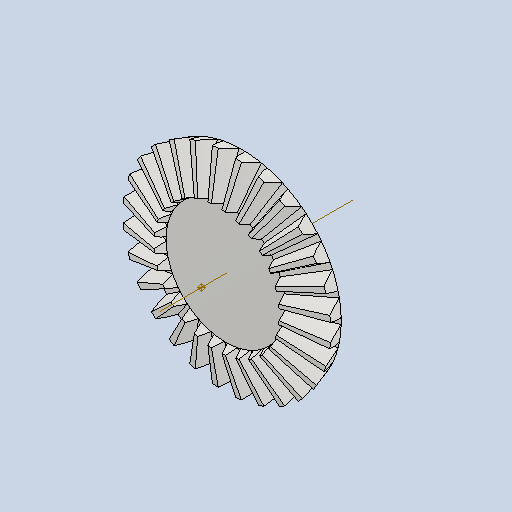
# Autodesk Inventor part: 베벨 기어2
Saved by Autodesk Inventor 2025.3 (Build 293356030, 356C)
## iProperties
Created: 2025-11-17
Part Number: 베벨 기어2
Material: Steel, Mild
Document SubType Name: Modeling
Designer: MSI
Categories: <?xml version="1.0" encoding="UTF-16"?> <MemberInstance><Categories><FamilyTemplate><FamilyTemplateParameter ValueType="xs:double" Id="1" ObjectReferenceKey="da_z" ObjectType="kUserParameterObject"/><FamilyTemplateParameter ValueType="xs:double" Id="2" ObjectReferenceKey="da_b" ObjectType="kUserParameterObject"/><FamilyTemplateParameter ValueType="xs:double" Id="3" ObjectReferenceKey="da_beta" ObjectType="kUserParameterObject"/><FamilyTemplateParameter ValueType="xs:double" Id="4" ObjectReferenceKey="da_dae" ObjectType="kUserParameterObject"/><FamilyTemplateParameter ValueType="xs:double" Id="5" ObjectReferenceKey="da_ve" ObjectType="kUserParameterObject"/><FamilyTemplateParameter ValueType="xs:double" Id="6" ObjectReferenceKey="da_omega" ObjectType="kUserParameterObject"/><FamilyTemplateParameter ValueType="xs:string" Id="7" ObjectReferenceKey="EAIAABAAAAAAHwAAAAAAAIAAAAAAAAAA" ObjectType="83914240" SubObjectId="SurfaceGeometry"/></FamilyTemplate><ParamToTemplateMap><ParamToTemplate CategoryParameter="//CategoryParameter[@InternalName='046C89C9-8512-4d59-83FE-43B91F4F132A']" TemplateParameter="1"/><ParamToTemplate CategoryParameter="//CategoryParameter[@InternalName='2552DF32-E462-4b46-AEBF-C6C7768E72AC']" TemplateParameter="2"/><ParamToTemplate CategoryParameter="//CategoryParameter[@InternalName='C9EE641D-15FC-4fae-A226-E94C4372FDD7']" TemplateParameter="3"/><ParamToTemplate><ParamToTemplate CategoryParameter="//CategoryParameter[@InternalName='00B6519A-459B-49c7-AD84-2E56D39A5744']" ConstantValue="-0.000000"/></ParamToTemplate><ParamToTemplate><ParamToTemplate CategoryParameter="//CategoryParameter[@InternalName='04B31F0E-C7A6-4894-AA32-9629BEFACF47']" ConstantValue="1.000000"/></ParamToTemplate><ParamToTemplate><ParamToTemplate CategoryParameter="//CategoryParameter[@InternalName='43CBEC2E-7847-49e7-A936-2F7889FCB2D9']" ConstantValue="0.200000"/></ParamToTemplate><ParamToTemplate><ParamToTemplate CategoryParameter="//CategoryParameter[@InternalName='B1EFC894-105D-4ebd-86BF-FA20ED196853']" ConstantValue="0.300000"/></ParamToTemplate><ParamToTemplate><ParamToTemplate CategoryParameter="//CategoryParameter[@InternalName='51175063-3D10-4879-93E8-6246FE8B403D']" ConstantValue="2060000000.000000"/></ParamToTemplate><ParamToTemplate><ParamToTemplate CategoryParameter="//CategoryParameter[@InternalName='A3A52E27-4454-46a9-B0BD-C932399B70AF']" ConstantValue="0.300000"/></ParamToTemplate><ParamToTemplate CategoryParameter="//CategoryParameter[@InternalName='2A200944-5A8C-41ca-B96E-8520D2E510F1']" TemplateParameter="4"/><ParamToTemplate><ParamToTemplate CategoryParameter="//CategoryParameter[@InternalName='1A637F62-92C8-44bc-B81F-10802510B579']" ConstantValue="3.445963"/></ParamToTemplate><ParamToTemplate CategoryParameter="//CategoryParameter[@InternalName='B52DD4BE-6863-48fb-BF58-89EF6F9EC65C']" TemplateParameter="5"/><ParamToTemplate><ParamToTemplate CategoryParameter="//CategoryParameter[@InternalName='3956BFF2-84D2-457d-93C2-9B0613DEBA67']" ConstantValue="0.427309"/></ParamToTemplate><ParamToTemplate CategoryParameter="//CategoryParameter[@InternalName='739CFA02-461B-4bf8-8049-181FCAD8B28F']" TemplateParameter="6"/><ParamToTemplate><ParamToTemplate CategoryParameter="//CategoryParameter[@InternalName='A27E999F-E2CE-4481-8A2A-EBF499C4C3C5']" ConstantValue="-0.000000"/></ParamToTemplate><ParamToTemplate><ParamToTemplate CategoryParameter="//CategoryParameter[@InternalName='9E1B4470-B2D3-4ff1-B813-535BB4CDF51A']" ConstantValue="3520000.000000"/></ParamToTemplate><ParamToTemplate><ParamToTemplate CategoryParameter="//CategoryParameter[@InternalName='F8452263-BFF6-458c-9FB1-07C4B99E95CD']" ConstantValue="11400000.000000"/></ParamToTemplate><ParamToTemplate><ParamToTemplate CategoryParameter="//CategoryParameter[@InternalName='3E3BB259-FD49-497f-8171-6EBC954A3479']" ConstantValue="2.000000"/></ParamToTemplate><ParamToTemplate CategoryParameter="//CategoryParameter[@InternalName='27C3BAF2-7550-4e4b-AE2C-0DB134B7D9B7']" TemplateParameter="7"/></ParamToTemplateMap><Category DisplayName="Gear" InternalName="DC85795E-93AB-48d5-8EEE-5A27447B64BD" Mnemonic="Gear"><CategoryParameter DisplayName="z" InternalName="046C89C9-8512-4d59-83FE-43B91F4F132A" Mnemonic="z"/><CategoryParameter DisplayName="b" InternalName="2552DF32-E462-4b46-AEBF-C6C7768E72AC" Mnemonic="b"/><CategoryParameter DisplayName="||b|" InternalName="C9EE641D-15FC-4fae-A226-E94C4372FDD7" Mnemonic="beta"/><CategoryParameter DisplayName="x" InternalName="00B6519A-459B-49c7-AD84-2E56D39A5744" Mnemonic="x"/><CategoryParameter DisplayName="a*" InternalName="04B31F0E-C7A6-4894-AA32-9629BEFACF47" Mnemonic="a"/><CategoryParameter DisplayName="c*" InternalName="43CBEC2E-7847-49e7-A936-2F7889FCB2D9" Mnemonic="c"/><CategoryParameter DisplayName="r|.f|*" InternalName="B1EFC894-105D-4ebd-86BF-FA20ED196853" Mnemonic="rf"/><CategoryParameter DisplayName="E" InternalName="51175063-3D10-4879-93E8-6246FE8B403D" Mnemonic="E"/><CategoryParameter DisplayName="||m|" InternalName="A3A52E27-4454-46a9-B0BD-C932399B70AF" Mnemonic="mi"/><Category DisplayName="BevelGear" InternalName="0C98F69A-0C2B-4791-B2FE-7691BB227E77" Mnemonic="BevelGear"><CategoryParameter DisplayName="d|.ae|" InternalName="2A200944-5A8C-41ca-B96E-8520D2E510F1" Mnemonic="dae"/><CategoryParameter DisplayName="d|.ai|" InternalName="1A637F62-92C8-44bc-B81F-10802510B579" Mnemonic="dai"/><CategoryParameter DisplayName="A|.e|" InternalName="B52DD4BE-6863-48fb-BF58-89EF6F9EC65C" Mnemonic="ve"/><CategoryParameter DisplayName="A|.i|" InternalName="3956BFF2-84D2-457d-93C2-9B0613DEBA67" Mnemonic="vi"/><CategoryParameter DisplayName="||S|" InternalName="739CFA02-461B-4bf8-8049-181FCAD8B28F" Mnemonic="omega"/><CategoryParameter DisplayName="x|.t|" InternalName="A27E999F-E2CE-4481-8A2A-EBF499C4C3C5" Mnemonic="xt"/><CategoryParameter DisplayName="||s||.Flim|" InternalName="9E1B4470-B2D3-4ff1-B813-535BB4CDF51A" Mnemonic="sFlim"/><CategoryParameter DisplayName="||s||.Hlim|" InternalName="F8452263-BFF6-458c-9FB1-07C4B99E95CD" Mnemonic="sHlim"/><CategoryParameter DisplayName="유형" InternalName="3E3BB259-FD49-497f-8171-6EBC954A3479" Mnemonic="type"/><CategoryParameter DisplayName="PitchDiameter" InternalName="27C3BAF2-7550-4e4b-AE2C-0DB134B7D9B7" Mnemonic="IDS_PITCHDIAM"/></Category></Category></Categories></MemberInstance>
Mass: 60.9118 g
Surface Area: 34.3074 cm^2
Volume: 7.7496 cm^3
Density: 7.86 g/cm^3
Appearance: Steel
CustomPartVersion: 1
Author: MSI
Autodesk Inventor part; units mm, degrees
ref_plane "메쉬 평면2" through (0, 0, 0) normal (0.9937122, 0.1119645, 0) x (0, 0, 1)
sketch "톱니 본체 스케치" plane through (0, 0, 0) normal (1, 0, 0) x (0, 1, 0)
  line L0 (0, 0) -> (27.265578, -11.284869) construction
  line L1 (27.265578, -11.284869) -> (28.612018, -7.095943)
  line L2 (28.612018, -7.095943) -> (0, 0) construction
  line L3 (28, -9) -> (0, 0) construction
  line L4 (16.419006, -6.795613) -> (17.229816, -4.273092)
  line L5 (27.265578, -11.284869) -> (16.419006, -6.795613)
  line L6 (28.612018, -7.095943) -> (17.229816, -4.273092)
  line L7 (0, -39.386751) -> (0, 6.564458)
  line L8 (0, -9) -> (28.612018, -9) construction
  dimension "d0" = 56
  dimension "d1" = 54.53116
  dimension "d2" = 57.22404
  dimension "d3" = 11.7
  dimension "d4" = 7.09594
  constraints: 16 end point, 4 point on line, 3 perpendicular, 2 collinear, 1 horizontal alignment, 1 vertical alignment
  measures "d0" diameter of L3.start L7
  measures "d1" diameter of L0.end L7
  measures "d2" diameter of L1.end L7
  measures "d3" distance between parallel lines of L1 L4
  measures "d4" vertical distance of L1.end L0.start
revolve "톱니 본체" add sketch "톱니 본체 스케치" angle 360 about axis through (0, 0, 0) along (0, 0, 1)
ref_plane "톱니 평면" through (0, 28, -9) normal (0, -0.9520286, 0.3060092) x (1, 0, 0)
sketch "시작 스케치" plane through (0, 28, -9) normal (0, -0.9520286, 0.3060092) x (1, 0, 0)
  line L0 (0, -23.505131) -> (0, 10.644758)
  arc A0 (-0.660229, -2.927998) -> (-3.024625, 3.271749) centre (-31.571304, -11.165819) ccw
  arc A1 (3.024625, 3.271749) -> (0.660229, -2.927998) centre (31.571304, -11.165819) ccw
  line L1 (-0.660229, -2.927998) -> (0.660229, -2.927998)
  arc A2 (3.024625, 3.271749) -> (-3.024625, 3.271749) centre (0, -91.500521) ccw
  dimension "d7" = 31.98994
  dimension "d8" = 31.5713
  dimension "d9" = 80.3347
  dimension "d57" = 94.82052
  dimension "d58" = 88.57252
  constraints: 6 point on circle, 3 centre point, 3 symmetric about line, 2 end point, 1 coincident, 1 perpendicular, 1 other
  measures "d7" radius of A0
  measures "d8" horizontal distance of point (0, -91.501) A0.centre
  measures "d9" vertical distance of point (0, -91.501) A0.centre
  measures "d57" radius of A2
  measures "d58" distance from line of A2.centre L1
ref_plane "끝 평면" through (0, 16.65182, -5.352371) normal (0, -0.9520286, 0.3060092) x (1, 0, 0)
sketch "끝 스케치" plane through (0, 16.65182, -5.352371) normal (0, -0.9520286, 0.3060092) x (1, 0, 0)
  line L0 (0, -15.35404) -> (0, 6.953444)
  arc A0 (-0.392643, -1.741305) -> (-1.798768, 1.945734) centre (-18.775702, -6.640401) ccw
  arc A1 (1.798768, 1.945734) -> (0.392643, -1.741305) centre (18.775702, -6.640401) ccw
  line L1 (-0.392643, -1.741305) -> (0.392643, -1.741305)
  arc A2 (1.798768, 1.945734) -> (-1.798768, 1.945734) centre (0, -54.416078) ccw
  dimension "d12" = 19.02467
  dimension "d15" = 18.7757
  dimension "d16" = 47.77568
  dimension "d59" = 56.39051
  dimension "d60" = 52.67477
  constraints: 6 point on circle, 3 centre point, 3 symmetric about line, 2 end point, 1 coincident, 1 other
  measures "d12" radius of A0
  measures "d15" horizontal distance of A0.centre point (0, -54.416)
  measures "d16" vertical distance of A0.centre point (0, -54.416)
  measures "d59" radius of A2
  measures "d60" distance from line of A2.centre L1
loft "Loft" cut profiles "시작 스케치", "끝 스케치"
pattern_circular "Circular Pattern" count 28 over 360 about axis through (0, 0, 0) along (0, 0, 1) of "Loft"
sketch3d "3D 스케치 오른쪽"
ref_plane "끝 평면 오른쪽" through (-3.200744, 16.341307, -5.352371) normal (0.182995, -0.9342758, 0.3060092) x (0.9813527, 0.1922159, 0)
sketch "끝 스케치 오른쪽" plane through (-3.200744, 16.341307, -5.352371) normal (0.182995, -0.9342758, 0.3060092) x (0.9813527, 0.1922159, 0)
  arc A0 (-0.392643, -1.741305) -> (-1.798768, 1.945734) centre (-18.775702, -6.640401) ccw
  line L0 (0, -67.117491) -> (0, 16.468068)
  arc A1 (1.798768, 1.945734) -> (0.392643, -1.741305) centre (18.775702, -6.640401) ccw
  line L1 (-0.392643, -1.741305) -> (0.392643, -1.741305)
  arc A2 (1.798768, 1.945734) -> (-1.798768, 1.945734) centre (0, -54.416078) ccw
  dimension "d70" = 18.7757
  dimension "d71" = 47.77568
  dimension "d72" = 19.02467
  dimension "d73" = 52.67477
  dimension "d74" = 56.39051
  constraints: 6 point on circle, 3 centre point, 3 symmetric about line, 2 end point, 1 coincident, 1 perpendicular, 1 other
  measures "d70" horizontal distance of A2.centre A0.centre
  measures "d71" vertical distance of point (0, -54.416) A0.centre
  measures "d72" radius of A0
  measures "d73" distance from line of point (0, -54.416) L1
  measures "d74" radius of A2
feature "로프트 오른쪽" [suppressed]
pattern_circular "원형 패턴 오른쪽" [suppressed]
sketch3d "3D 스케치 왼쪽"
ref_plane "끝 평면 왼쪽" through (3.32113, 16.341307, -5.46163) normal (-0.1892704, -0.9312872, 0.311257) x (0.9799662, -0.1991637, 0)
sketch "끝 스케치 왼쪽" plane through (3.32113, 16.341307, -5.46163) normal (-0.1892704, -0.9312872, 0.311257) x (0.9799662, -0.1991637, 0)
  line L0 (0, -68.172924) -> (0, 17.623134)
  arc A0 (-0.392643, -1.643977) -> (-1.798768, 2.043061) centre (-18.775702, -6.543073) ccw
  arc A1 (1.798768, 2.043061) -> (0.392643, -1.643977) centre (18.775702, -6.543073) ccw
  line L1 (-0.392643, -1.643977) -> (0.392643, -1.643977)
  ellipse E0 centre (0, -4.06083) end of major axis (17.229816, -4.06083) minor radius 5.362901
  arc A2 (1.798768, 2.043061) -> (-1.798768, 2.043061) centre (0, -54.318751) ccw
  dimension "d56" = 5.3629
  dimension "d30" = 19.02467
  dimension "d31" = 18.7757
  dimension "d32" = 47.77568
  dimension "d61" = 56.39051
  dimension "d62" = 52.67477
  constraints: 6 point on circle, 3 centre point, 3 symmetric about line, 2 end point, 1 coincident, 2 other
  measures "d30" radius of A0
  measures "d31" horizontal distance of point (0, -54.319) A0.centre
  measures "d32" vertical distance of A0.centre point (0, -54.319)
  measures "d61" radius of A2
  measures "d62" distance from line of point (0, -54.319) L1
feature "로프트 왼쪽" [suppressed]
pattern_circular "원형 패턴 왼쪽" [suppressed]
sketch "본체 스케치" plane through (0, 0, 0) normal (1, 0, 0) x (0, 1, 0)
  line L0 (0, -35.037536) -> (0, -19.530831)
  line L1 (27.265578, -11.284869) -> (16.419006, -6.795613)
  line L2 (16.419006, -6.795613) -> (0, -6.795613)
  line L3 (27.265578, -11.284869) -> (0, -11.284869)
  constraints: 4 end point, 2 perpendicular, 2 point on line
sketch "본체 스케치 outline for 본체 고정" plane through (0, 0, 0) normal (1, 0, 0) x (0, 1, 0)
  line L0 (0, -11.284869) -> (27.265578, -11.284869)
  line L1 (0, -6.795613) -> (0, -11.284869)
  line L2 (16.419006, -6.795613) -> (0, -6.795613)
  line L3 (27.265578, -11.284869) -> (16.419006, -6.795613)
revolve "본체 고정" add sketch "본체 스케치 outline for 본체 고정" angle 360 about axis through (0, 0, 0) along (0, 0, 1)
sketch "Sketch6" plane through (0, 0, 0) normal (1, 0, 0) x (0, 1, 0)
  line L0 (28, -9) -> (0, 0)
  line L1 (0, -37.799919) -> (0, 6.299986)
surface revolve "피치 지름" sketch "Sketch6" angle 360 about axis through (0, 0, 0) along (0, 0, 1) shown no curves L0
equation "\"d0\" = da_de"
equation "\"d1\" = da_dfe"
equation "\"d2\" = da_dae"
equation "\"d3\" = da_b"
equation "\"d4\" = da_ve"
equation "\"d7\" = fd_rr"
equation "\"d8\" = fd_x"
equation "\"d9\" = fd_y"
equation "\"d57\" = 0.5 * fd_dva + 0.3 * da_he"
equation "\"d58\" = 0.5 * fd_dva - 1.12 * da_he"
equation "\"da_teethtype\" = 0"
equation "\"da_b\" = 11.7"
equation "\"da_de\" = 56"
equation "\"da_dae\" = 57.22404"
equation "\"da_dfe\" = 54.53116"
equation "\"da_le\" = 29.41088"
equation "\"da_omega\" = 90deg"
equation "\"da_beta\" = 0"
equation "\"da_delta\" = 72.181111deg"
equation "\"da_alpha\" = 20deg"
equation "\"da_he\" = 4.4"
equation "\"da_ve\" = 7.09594"
equation "\"da_zv\" = 91.500523"
equation "\"fd_loft\" = da_b + 0.05 * da_he"
equation "\"fd_x\" = fd_x1 + fd_x2"
equation "\"fd_y\" = fd_y1 - fd_y2"
equation "\"fd_dd\" = fd_dva - 0.8 * da_he"
equation "\"da_dvw\" = 183.00105"
equation "\"d11\" = fd_loft"
equation "\"da_dm\" = 44.86127"
equation "\"da_x\" = 0"
equation "\"da_m\" = 2"
equation "\"d50\" = da_omega"
equation "\"fd_rr\" = 31.98994"
equation "\"fd_dva\" = 187.001046"
equation "\"fd_x1\" = 1.58817"
equation "\"fd_x2\" = 29.983134"
equation "\"fd_y1\" = 91.486739"
equation "\"fd_y2\" = 11.152036"
body "Solid1"
body "Srf1"
